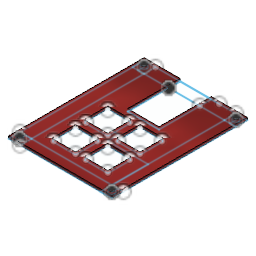
shauryapad (Autodesk Fusion 360 archive; units mm, degrees)
design "Case"
part number: 2025-11-20-10-30-27-807
Autodesk Fusion 360 part; units mm, degrees
sketch "plate-2025-11-20T02_26_56.904Z" plane through (0, 0, 0) normal (0, 1, 0) x (1, 0, 0)
sketch "plate-2025-11-20T02_26_56.904Z (1)" plane through (0, 0, 0) normal (0, 1, 0) x (1, 0, 0)
  line L0 (3.025, -2.525) -> (16.025, -2.5274)
  line L1 (3.025, -16.525) -> (16.025, -16.525)
  line L2 (2.525, -3.025) -> (2.525, -16.025)
  line L3 (16.5157, -3.025) -> (16.5157, -16.025)
  arc A0 (3.025, -2.525) -> (2.525, -3.025) centre (3.025, -3.025) ccw
  arc A1 (16.5157, -3.025) -> (16.025, -2.5274) centre (16.0207, -3.0224) ccw
  arc A2 (2.525, -16.025) -> (3.025, -16.525) centre (3.025, -16.025) ccw
  arc A3 (16.025, -16.525) -> (16.5157, -16.025) centre (16.0194, -16.0287) ccw
  line L4 (22.105, -2.525) -> (35.105, -2.525)
  line L5 (22.105, -16.525) -> (35.105, -16.525)
  line L6 (21.5957, -3.025) -> (21.5957, -16.025)
  line L7 (35.605, -3.025) -> (35.605, -16.025)
  arc A4 (22.105, -2.525) -> (21.5957, -3.025) centre (22.1001, -3.0294) ccw
  arc A5 (35.605, -3.025) -> (35.105, -2.525) centre (35.105, -3.025) ccw
  arc A6 (21.5957, -16.025) -> (22.105, -16.525) centre (22.0993, -16.0214) ccw
  arc A7 (35.105, -16.525) -> (35.605, -16.025) centre (35.105, -16.025) ccw
  line L8 (3.025, -21.605) -> (16.025, -21.605)
  line L9 (3.025, -35.605) -> (16.025, -35.605)
  line L10 (2.525, -22.105) -> (2.525, -35.105)
  line L11 (16.525, -22.105) -> (16.525, -35.105)
  arc A8 (3.025, -21.605) -> (2.525, -22.105) centre (3.025, -22.105) ccw
  arc A9 (16.525, -22.105) -> (16.025, -21.605) centre (16.025, -22.105) ccw
  arc A10 (2.525, -35.105) -> (3.025, -35.605) centre (3.025, -35.105) ccw
  arc A11 (16.025, -35.605) -> (16.525, -35.105) centre (16.025, -35.105) ccw
  line L12 (22.105, -21.605) -> (35.105, -21.605)
  line L13 (22.105, -35.605) -> (35.105, -35.605)
  line L14 (21.605, -22.105) -> (21.605, -35.105)
  line L15 (35.605, -22.105) -> (35.605, -35.105)
  arc A12 (22.105, -21.605) -> (21.605, -22.105) centre (22.105, -22.105) ccw
  arc A13 (35.605, -22.105) -> (35.105, -21.605) centre (35.105, -22.105) ccw
  arc A14 (21.605, -35.105) -> (22.105, -35.605) centre (22.105, -35.105) ccw
  arc A15 (35.105, -35.605) -> (35.605, -35.105) centre (35.105, -35.105) ccw
  line L16 (16.5157, -12.518) -> (19.0557, -12.518)
  line L17 (19.0557, -12.518) -> (19.0557, -19)
  line L18 (19.0557, -19) -> (42.8682, -19)
  line L19 (42.8682, -19) -> (42.8682, -40.431)
  line L20 (42.8682, -40.431) -> (-4.7568, -40.431)
  line L21 (-4.7568, -40.431) -> (-4.7568, 26.244)
  line L22 (-4.7568, 26.244) -> (42.8682, 26.244)
  line L23 (42.8682, 26.244) -> (42.8682, -40.431)
  line L24 (9.8057, 26.244) -> (28.3057, 26.244)
  line L25 (-4.7568, 26.244) -> (-11.5568, 26.244)
  line L26 (-4.7568, 26.244) -> (-4.7568, 33.044)
  line L27 (42.8682, 26.244) -> (42.8682, 33.044)
  line L28 (42.8682, 26.244) -> (49.6682, 26.244)
  line L29 (42.8682, -40.431) -> (42.8682, -47.231)
  line L30 (42.8682, -40.431) -> (49.6682, -40.431)
  line L31 (-4.7568, -40.431) -> (-4.7568, -47.231)
  line L32 (-4.7568, -40.431) -> (-11.5568, -40.431)
  line L33 (-11.5568, 26.244) -> (-11.5568, 33.044)
  line L34 (42.8682, -47.231) -> (49.6682, -47.231)
  line L35 (49.6682, -47.231) -> (-11.5568, -47.231)
  line L36 (-11.5568, -47.231) -> (-11.5568, 33.044)
  line L37 (-11.5568, 33.044) -> (49.6682, 33.044)
  line L38 (49.6682, 33.044) -> (49.6682, -47.231)
  line L39 (9.8057, 26.244) -> (9.8057, 33.044)
  line L40 (9.8057, 33.044) -> (33, 33.044)
  line L41 (9.8057, 2.044) -> (9.8057, 33.044)
  line L42 (9.8057, 2.044) -> (28.3057, 2.044)
  line L43 (28.3057, 2.044) -> (9.8057, 2.044)
  line L44 (9.8057, 2.044) -> (9.8057, 33.044)
  line L45 (9.8057, 33.044) -> (28.3057, 33.044)
  line L46 (28.3057, 33.044) -> (28.3057, 2.044)
  line L47 (-4.7568, -40.431) -> (-8.2928, -40.431)
  line L48 (-8.2928, -40.431) -> (-8.2928, -43.967)
  line L49 (-4.7568, 26.244) -> (-8.2928, 26.244)
  line L50 (-8.2928, 26.244) -> (-8.2928, 29.78)
  line L51 (49.6682, 26.244) -> (46.1322, 26.244)
  line L52 (46.1322, 26.244) -> (46.1322, 29.78)
  line L53 (42.8682, -40.431) -> (46.4042, -40.431)
  line L54 (46.4042, -40.431) -> (46.4042, -43.967)
  circle A16 centre (-8.2928, -43.967) radius 1.7
  circle A17 centre (-8.2928, 29.78) radius 1.7
  circle A18 centre (46.1322, 29.78) radius 1.7
  circle A19 centre (46.4042, -43.967) radius 1.7
  point P0 (9.8057, 26.244)
  dimension "d6" = 5.08
  dimension "d7" = 5.08
  dimension "d8" = 5.08
  dimension "d9" = 5.08
  dimension "d10" = 2.54
  dimension "d12" = 23.8125
  dimension "d13" = 21.431
  dimension "d14" = 66.675
  dimension "d15" = 47.625
  dimension "d16" = 14.5625
  dimension "d18" = 21.431
  dimension "d20" = 6.8
  dimension "d21" = 6.8
  dimension "d22" = 6.8
  dimension "d23" = 6.8
  dimension "d24" = 6.8
  dimension "d25" = 6.8
  dimension "d26" = 6.8
  dimension "d27" = 6.8
  dimension "d28" = 6.8
  dimension "d29" = 6.8
  dimension "d30" = 31
  dimension "d32" = 18.5
  dimension "d33" = 3.536
  dimension "d34" = 3.536
  dimension "d35" = 3.536
  dimension "d36" = 3.536
  dimension "d37" = 3.536
  dimension "d38" = 3.536
  dimension "d39" = 3.536
  dimension "d40" = 3.536
  dimension "d41" = 3.4
  dimension "d42" = 3.4
  dimension "d43" = 3.4
  dimension "d44" = 3.4
  constraint coincident L3 L16.start
  constraint perpendicular L3 L16
  constraint perpendicular L16 L17
  constraint perpendicular L17 L18
  constraint perpendicular L18 L19
  constraint horizontal L20
  constraint vertical L21
  constraint horizontal L22
  constraint vertical L23
  constraint coincident L22 P0
  constraint horizontal L24
  constraint coincident P0 L24.start
  constraint perpendicular L21 L25
  constraint perpendicular L22 L26
  constraint perpendicular L22 L27
  constraint perpendicular L27 L28
  constraint perpendicular L20 L29
  constraint perpendicular L19 L30
  constraint perpendicular L20 L31
  constraint perpendicular L31 L32
  constraint perpendicular L25 L33
  constraint perpendicular L29 L34
  constraint horizontal L35
  constraint vertical L36
  constraint horizontal L37
  constraint vertical L38
  constraint coincident L37 L39.end
  constraint perpendicular L37 L39
  constraint horizontal L40
  constraint vertical L41
  constraint perpendicular L41 L42
  constraint horizontal L43
  constraint vertical L44
  constraint horizontal L45
  constraint vertical L46
  constraint perpendicular L31 L47
  constraint perpendicular L32 L48
  constraint perpendicular L26 L49
  constraint perpendicular L25 L50
  constraint perpendicular L38 L51
  constraint perpendicular L51 L52
  constraint perpendicular L23 L53
  constraint perpendicular L53 L54
  constraint coincident L48.end A16.centre
  constraint coincident L50.end A17.centre
  constraint coincident L52.end A18.centre
  constraint coincident L54.end A19.centre
  measures "d6" distance of L5 L12
  measures "d7" distance of L1 L8
  measures "d8" distance of L3 L6
  measures "d9" distance of L11 L14
  measures "d10" distance of L16.start L16.end
  measures "d12" distance of L17.end L18.end
  measures "d13" distance of L18.end L19.end
  measures "d14" distance of L19.end L22.end
  measures "d15" distance of L19.end L20.end
  measures "d16" distance of L21.end P0
  measures "d18" distance of L17.end L20
  measures "d20" distance of L21.end L25.end
  measures "d21" distance of L21.end L26.end
  measures "d22" distance of L22.end L27.end
  measures "d23" distance of L22.end L28.end
  measures "d24" distance of L19.end L29.end
  measures "d25" distance of L19.end L30.end
  measures "d26" distance of L20.end L31.end
  measures "d27" distance of L20.end L32.end
  measures "d28" distance of L25.end L33.end
  measures "d29" distance of L29.end L34.end
  measures "d30" distance of L39.end L41.start
  measures "d32" distance of L41.start L42.end
  measures "d33" distance of L20.end L47.end
  measures "d34" distance of L47.end L48.end
  measures "d35" distance of L21.end L49.end
  measures "d36" distance of L49.end L50.end
  measures "d37" distance of L28.end L51.end
  measures "d38" distance of L51.end L52.end
  measures "d39" distance of L19.end L53.end
  measures "d40" distance of L53.end L54.end
  measures "d41" diameter of A16
  measures "d42" diameter of A17
  measures "d43" diameter of A18
  measures "d44" diameter of A19
extrude "Extrude1" add sketch "plate-2025-11-20T02_26_56.904Z (1)" along normal blind 1.5 contours L19 L20 L21 L22 L23 L41 L42 L43 L44 L46 makes body 1
extrude "Extrude2" add sketch "plate-2025-11-20T02_26_56.904Z (1)" along normal blind 1.5 separate body contours L19 L23 L28 L30 L38 L51 L53 | L29 L30 L34 L35 L38 L53 | L27 L28 L37 L38 L51 makes body 2
extrude "Extrude3" add sketch "plate-2025-11-20T02_26_56.904Z (1)" along normal blind 1.5 contours L20 L29 L31 L35 | L31 L32 L35 L36 L47 bodies 1 2
extrude "Extrude4" add sketch "plate-2025-11-20T02_26_56.904Z (1)" along normal blind 1.5 contours L21 L25 L32 L36 L47 L49 | L25 L26 L33 L36 L37 L49 bodies 1
extrude "Extrude5" add sketch "plate-2025-11-20T02_26_56.904Z (1)" along normal blind 1.5 contours L22 L26 L37 L39 L41 L44 bodies 1
extrude "Extrude6" add sketch "plate-2025-11-20T02_26_56.904Z (1)" along normal blind 1.5 contours L22 L27 L37 L40 L46 bodies 1
equation "d12 = ( 47.625 / 2 ) * 1 mm"
